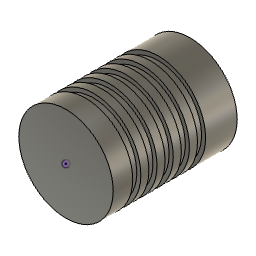
can (Autodesk Fusion 360 design; units mm, degrees)
Autodesk Fusion 360 part; units mm, degrees
sketch "Sketch1" plane through (0, 0, 0) normal (0, 0, 1) x (1, 0, 0)
sketch "Sketch2" plane through (0, 0, 0) normal (0, 0, 1) x (1, 0, 0)
sketch "Sketch3" plane through (0, 0, 0) normal (0, 0, 1) x (1, 0, 0)
  line L0 (0, 0) -> (0, 153.12)
  line L1 (-58.235, 153.12) -> (-58.235, 114.12)
  line L2 (-58.235, 114.12) -> (-53.235, 114.12)
  line L3 (-53.235, 114.12) -> (-53.235, 104.12)
  line L4 (-53.235, 104.12) -> (-58.235, 104.12)
  line L5 (-58.235, 104.12) -> (-58.235, 94.12)
  line L6 (-58.235, 94.12) -> (-53.235, 94.12)
  line L7 (-53.235, 94.12) -> (-53.235, 84.12)
  line L8 (-53.235, 84.12) -> (-58.235, 84.12)
  line L9 (-58.235, 84.12) -> (-58.235, 74.12)
  line L10 (-58.235, 74.12) -> (-53.235, 74.12)
  line L11 (-53.235, 74.12) -> (-53.235, 64.12)
  line L12 (-53.235, 64.12) -> (-58.235, 64.12)
  line L13 (-58.235, 64.12) -> (-58.235, 54.12)
  line L14 (-58.235, 54.12) -> (-53.235, 54.12)
  line L15 (-53.235, 54.12) -> (-53.235, 44.12)
  line L16 (-53.235, 44.12) -> (-58.235, 44.12)
  line L17 (-58.235, 44.12) -> (-58.235, 34.12)
  line L18 (-58.235, 34.12) -> (-53.235, 34.12)
  line L19 (-53.235, 34.12) -> (-53.235, 24.12)
  line L20 (-53.235, 24.12) -> (-58.235, 24.12)
  line L21 (-58.235, 24.12) -> (-58.235, 5.0228)
  line L22 (-58.235, 5.0228) -> (-58.235, 0)
  line L23 (-58.235, 153.12) -> (0, 153.12)
  line L24 (-58.235, 0) -> (0, 0)
  dimension "d4" = 153.12
  dimension "d5" = 58.235
  dimension "d6" = 39
  dimension "d7" = 5
  dimension "d8" = 10
  dimension "d9" = 5
  dimension "d10" = 10
  dimension "d11" = 5
  dimension "d12" = 10
  dimension "d13" = 5
  dimension "d14" = 10
  dimension "d15" = 5
  dimension "d16" = 10
  dimension "d17" = 5
  dimension "d18" = 10
  dimension "d19" = 5
  dimension "d20" = 10
  dimension "d21" = 5
  dimension "d22" = 10
  dimension "d23" = 5
  dimension "d24" = 10
  dimension "d25" = 5
  constraint coincident L0.start L24.end
  constraint vertical L0
  constraint vertical L1
  constraint perpendicular L1 L2
  constraint perpendicular L2 L3
  constraint perpendicular L3 L4
  constraint perpendicular L4 L5
  constraint perpendicular L5 L6
  constraint perpendicular L6 L7
  constraint perpendicular L7 L8
  constraint perpendicular L8 L9
  constraint perpendicular L9 L10
  constraint perpendicular L10 L11
  constraint perpendicular L11 L12
  constraint perpendicular L12 L13
  constraint perpendicular L13 L14
  constraint perpendicular L14 L15
  constraint perpendicular L15 L16
  constraint perpendicular L16 L17
  constraint perpendicular L17 L18
  constraint perpendicular L18 L19
  constraint perpendicular L19 L20
  constraint perpendicular L20 L21
  constraint parallel L21 L22
  constraint perpendicular L0 L23
  constraint perpendicular L0 L24
  measures "d4" distance of L0.start L0.end
  measures "d5" distance of L0.end L1.start
  measures "d6" distance of L1.end L1.start
  measures "d7" distance of L1.end L2.end
  measures "d8" distance of L2.end L3.end
  measures "d9" distance of L3.end L4.end
  measures "d10" distance of L4.end L5.end
  measures "d11" distance of L5.end L6.end
  measures "d12" distance of L6.end L7.end
  measures "d13" distance of L7.end L8.end
  measures "d14" distance of L8.end L9.end
  measures "d15" distance of L9.end L10.end
  measures "d16" distance of L10.end L11.end
  measures "d17" distance of L11.end L12.end
  measures "d18" distance of L12.end L13.end
  measures "d19" distance of L13.end L14.end
  measures "d20" distance of L14.end L15.end
  measures "d21" distance of L15.end L16.end
  measures "d22" distance of L16.end L17.end
  measures "d23" distance of L17.end L18.end
  measures "d24" distance of L18.end L19.end
  measures "d25" distance of L19.end L20.end
revolve "Revolve1" add sketch "Sketch3" angle 360 about axis through (0, 0, 0) along (0, 1, 0)
